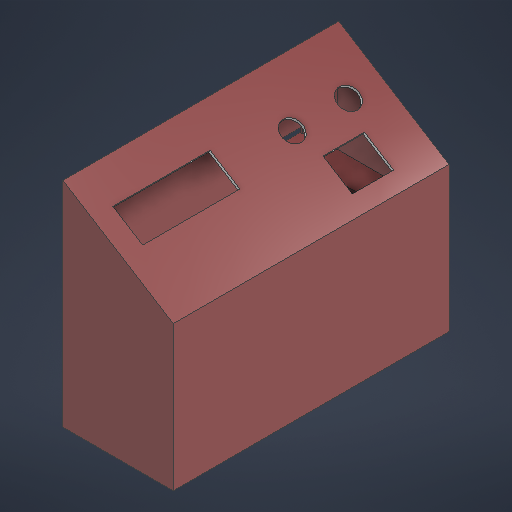
# Autodesk Inventor part: Housing og Buttons & LCD
Saved by Autodesk Inventor 2026.2 (Build 302298010, 298A)
## iProperties
Created: 2026-05-24
Part Number: Housing og Buttons & LCD
Material: Generic
Document SubType Name: Modeling
Designer: lenovo
Density: 1 g/cm^3
Appearance: Default
Author: lenovo
Autodesk Inventor part; units mm, degrees
ref_plane "YZ Plane" through (0, 0, 0) normal (1, 0, 0) x (0, 1, 0)
ref_plane "XZ Plane" through (0, 0, 0) normal (0, 1, 0) x (-1, 0, 0)
ref_plane "XY Plane" through (0, 0, 0) normal (0, 0, 1) x (1, 0, 0)
sketch "Sketch1" plane through (0, 0, 0) normal (0, 0, 1) x (1, 0, 0)
  line L0 (0, 0) -> (80, 0)
  line L1 (0, 0) -> (0, 155)
  line L2 (80, 0) -> (80, 105)
  line L3 (80, 105) -> (0, 155)
  dimension "d0" = 80
  dimension "d1" = 155
  dimension "d2" = 105
  constraints: 8 end point, 1 horizontal, 1 parallel, 1 perpendicular
  measures "d0" distance of L0.start L0.end
  measures "d1" distance of L0.start L1.end
  measures "d2" distance of L0.end L2.end
extrude "Extrusion1" add sketch "Sketch1" along normal blind 200
sketch "Sketch3" plane through (0, 0, 200) normal (0, 0, 1) x (1, 0, 0)
  line L0 (2, 0) -> (2, 151.3915)
  line L1 (80, 0) -> (80, 105) projected
  line L2 (78, 0) -> (78, 103.8915)
  line L3 (80, 105) -> (0, 155) projected
  line L4 (2, 151.3915) -> (78, 103.8915)
  line L5 (0, 0) -> (80, 0) projected
  line L6 (2, 0) -> (78, 0)
  line L7 (0, 155) -> (0, 0) projected
  dimension "d23" = 2
  dimension "d24" = 2
  dimension "d25" = 2
  constraints: 8 end point, 2 point on line, 1 parallel, 1 vertical
  measures "d23" distance between parallel lines of L3 L4
  measures "d24" distance between parallel lines of L7 L0
  measures "d25" distance between parallel lines of L1 L2
extrude "Extrusion3" cut sketch "Sketch3" against normal blind 197 contours L0 L4 L2 L5
extrude "Extrusion4" add sketch "Sketch3" against normal blind 3 contours L0 L4 L2 L5
sketch "Sketch4" plane through (0, 0, 0) normal (-1, 0, 0) x (0, 0, 1)
  line L0 (0, 155) -> (0, 0) projected
  line L1 (0, 155) -> (0, 105)
  line L2 (28, 99.083) -> (42, 99.083)
  line L3 (42, 99.083) -> (42, 104)
  line L4 (42, 104) -> (28, 104)
  line L5 (28, 104) -> (28, 99.083)
  line L6 (28, 99.083) -> (42, 99.083)
  line L7 (0, 155) -> (0, 105)
  line L8 (0, 155) -> (200, 155) projected
  line L9 (28, 99.083) -> (42, 99.083)
  point P0 (28, 101.5415)
  dimension "d47" = 28
  dimension "d48" = 51
  constraints: 16 end point, 2 perpendicular, 1 collinear, 1 midpoint, 1 point on line
  measures "d47" distance from line of L0 point (28, 101.542)
  measures "d48" distance between parallel lines of L8 L4
extrude "Extrusion5" cut sketch "Sketch4" against normal blind 10
sketch "Sketch5" plane through (2, 0, 3) normal (1, 0, 0) x (0, 0, -1)
  line L0 (-25, 99.083) -> (-39, 99.083) projected
  line L1 (-25, 99.083) -> (-22, 99.083)
  line L2 (-39, 99.083) -> (-42, 99.083)
  line L3 (-42, 99.083) -> (-22, 99.083)
  line L4 (-22, 99.083) -> (-22, 96.083)
  line L5 (-22, 96.083) -> (-42, 96.083)
  line L6 (-42, 96.083) -> (-42, 99.083)
  point P0 (3, 0)
  dimension "d42" = 3
  dimension "d43" = 3
  dimension "d44" = 3
  constraints: 12 end point, 3 perpendicular, 2 horizontal, 1 collinear
  measures "d42" distance of L0.start L1.end
  measures "d43" distance of L0.end L2.end
  measures "d44" distance of L1.end L4.end
extrude "Extrusion6" add sketch "Sketch5" along normal blind 60
sketch "Sketch6" plane through (0, 155, 200) normal (0.53, 0.848, 0) x (0.848, -0.53, 0)
  line L0 (25, 15) -> (50.5, 15)
  line L1 (50.5, 15) -> (50.5, 85.5)
  line L2 (50.5, 85.5) -> (25, 85.5)
  line L3 (25, 85.5) -> (25, 15)
  line L4 (94.3398, 0) -> (0, 0) projected
  line L5 (0, 200) -> (0, 0) projected
  line L6 (32.9219, 175) -> (83.8018, 175) projected
  circle A0 centre (37.75, 175) radius 7.75
  circle A1 centre (37.75, 134.2821) radius 7.75
  line L7 (82.3488, 140) -> (57.3488, 140)
  line L8 (57.3488, 140) -> (57.3488, 170)
  line L9 (57.3488, 170) -> (82.3488, 170)
  line L10 (82.3488, 170) -> (82.3488, 140)
  line L11 (31.3319, 155) -> (82.2118, 155) projected
  line L12 (82.3488, 140) -> (57.3488, 170) construction
  line L13 (57.3488, 140) -> (82.3488, 170) construction
  point P0 (82.1498, 200)
  point P1 (69.8488, 155)
  dimension "d49" = 25.5
  dimension "d50" = 70.5
  dimension "d51" = 15
  dimension "d52" = 25
  dimension "d53" = 15.5
  dimension "d54" = 15.5
  dimension "d55" = 25
  dimension "d56" = 30
  constraints: 20 end point, 4 parallel, 2 centre point, 2 horizontal, 2 midpoint, 2 perpendicular, 2 point on line
  measures "d49" distance of L2.end L1.end
  measures "d50" distance of L1.end L0.end
  measures "d51" distance between parallel lines of L4 L0
  measures "d52" distance between parallel lines of L5 L3
  measures "d53" diameter of A0
  measures "d54" diameter of A1
  measures "d55" distance of L8.end L9.end
  measures "d56" distance of L7.end L8.end
extrude "Extrusion7" cut sketch "Sketch6" against normal blind 10
body "Solid1"
